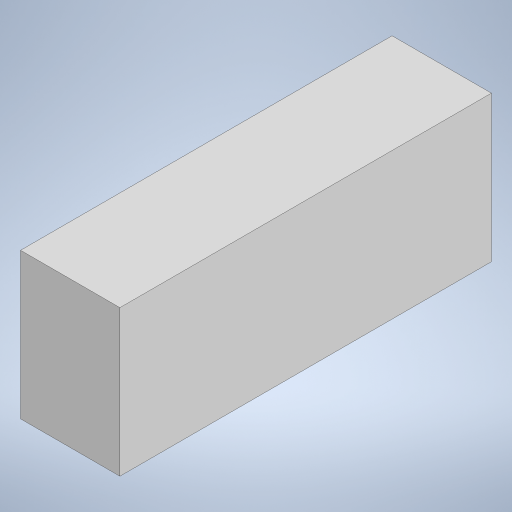
# Autodesk Inventor part: LC-LC-Coupler
Saved by Autodesk Inventor 2024 (Build 280153000, 153)
## iProperties
Created: 2025-02-14
Part Number: LC-LC-Coupler
Material: Generic
Document SubType Name: Modeling
Designer: phdgc
Density: 1 g/cm^3
Appearance: Default
Author: phdgc
Autodesk Inventor part; units mm, degrees
ref_plane "YZ Plane" through (0, 0, 0) normal (1, 0, 0) x (0, 1, 0)
ref_plane "XZ Plane" through (0, 0, 0) normal (0, 1, 0) x (-1, 0, 0)
ref_plane "XY Plane" through (0, 0, 0) normal (0, 0, 1) x (1, 0, 0)
sketch "Sketch1" plane through (0, 0, 0) normal (0, 0, 1) x (1, 0, 0)
  line L0 (0, 0) -> (6.86, 0)
  line L1 (6.86, 0) -> (6.86, 10.08)
  line L2 (6.86, 10.08) -> (0, 10.08)
  line L3 (0, 10.08) -> (0, 0)
  circle A0 centre (3.43, 5.04) radius 1.5
  dimension "d0" = 6.86
  dimension "d1" = 10.08
  dimension "d4" = 3
  constraints: 8 end point, 2 parallel, 1 centre point, 1 horizontal, 1 perpendicular
  measures "d0" distance of L2.end L1.end
  measures "d1" distance of L1.end L0.end
  measures "d4" diameter of A0
extrude "Extrusion1" add sketch "Sketch1" along normal blind 25.65 contours L3 L2 L1 L0 | A0
body "Solid1"
